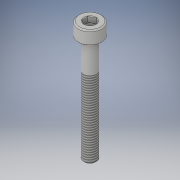
# Autodesk Inventor part: DIN-912 - M3x25(F)
Saved by Autodesk Inventor 2019 (Build 230136000, 136)
## iProperties
Created: 2023-04-07
Part Number: DIN-912 - M3x25(F)
Material: Generic
Catalog Web Link: www.cadenas.de
Description: DIN-912-Cylinder screw
Vendor: FESTO
Document SubType Name: Modeling
Designer: psAdmin
Manufacturer: FESTO
Mass: 0.238597 g
Surface Area: 3.40249 cm^2
Volume: 0.238597 cm^3
Density: 1 g/cm^3
Appearance: PSOLRGB-175-175-175
Category: PARTsolutions
Company: FESTO
Title: DIN-912 - M3x25(F)
Author: Cadenas PARTsolutions
Comments: Cylinder screw
PSOL_IDENT_0: {$CADENAS_DATA/23d-libs/festo/zyl_zubeh/d912/din_912.prj},178 {VTYP=3D},{NB=DIN-912 - M3x25(F)},{LIN
PSOL_IDENT_1: A=DIN-912 - M3x25(F)},{NN=DIN-912},{DATE=25.11.2021 14:13:45},{GEOMDATE=25.11.2021 14:12:35},{VERSIO
PSOL_IDENT_2: N=},{LINEID=160},{WBVAR=},{WBNUMERIC=}  {NB=DIN-912 - M3x25(F)},{LINA=DIN-912 - M3x25(F)},{KT=X},{ID
PSOL_IDENT_3: NR=},{GEW=M3},{DG=3.000},{P=0.500},{L=25.000},{B=18.000},{FORM=0},{GKD=2.387},{DK=5.500},{DADIN=3.60
PSOL_IDENT_4: 0},{DS=3.000},{E=2.870},{LF=0.510},{K=3.000},{R=0.120},{S=2.500},{T=1.300},{V=0.300},{DW=5.070},{W=1
PSOL_IDENT_5: .150},{NENN=M3x25},{DA=3.1},{BL=18}
NB: DIN-912 - M3x25(F)
NN: DIN-912
NT: Cylinder screw
NBSYN: DIN-912 - $NENN.(F)
LINA: DIN-912 - M3x25(F)
CATALOG: Festo
ROWDESC: M3x25
GEW: M3
DG: 3
P: 0.5
L: 25
B: 18
FORM: 0
GKD: 2.387
DK: 5.5
DADIN: 3.6
DS: 3
E: 2.87
LF: 0.51
K: 3
R: 0.12
S: 2.5
T: 1.3
V: 0.3
DW: 5.07
W: 1.15
SUPPLIER: FESTO
ARTICLENO: DIN-912 - M3x25(F)
BOMINFO: DIN-912 - M3x25(F)
CREATOR: CADENAS GmbH
Autodesk Inventor part; units mm, degrees
sketch "Sketch_1" plane through (0, 0, 0) normal (0, 0, 1) x (1, 0, 0)
  line L0 (0, -25) -> (0, 3)
  line L1 (0, 0.9783) -> (1.25, 1.7)
  line L2 (1.25, 1.7) -> (1.25, 2.8066)
  line L3 (1.25, 2.8066) -> (1.4434, 3)
  line L4 (1.4434, 3) -> (2.45, 3)
  line L5 (2.45, 3) -> (2.75, 2.7)
  line L6 (2.75, 2.7) -> (2.75, 0.075)
  line L7 (2.75, 0.075) -> (2.675, 0)
  line L8 (2.675, 0) -> (1.55, 0)
  line L9 (1.55, 0) -> (1.5, -0.51)
  line L10 (1.5, -0.51) -> (1.5, -24.6935)
  line L11 (1.5, -24.6935) -> (1.1935, -25)
  line L12 (1.1935, -25) -> (0, -25)
  line L13 (0, -25) -> (0, 0.9783)
  constraints: 28 end point
revolve "Revolution1" add sketch "Sketch_1" angle 360 about axis through (0, -25, 0) along (0, -1, 0)
thread "Thread1" size "M3x0.5" class "6g" standard "ISO Metric profile" length 17.6935
sketch "Sketch_2" plane through (0, 3, 0) normal (0, 1, 0) x (1, 0, 0)
  line L0 (-1.25, -0.7217) -> (0, -1.4434)
  line L1 (0, -1.4434) -> (1.25, -0.7217)
  line L2 (1.25, -0.7217) -> (1.25, 0.7217)
  line L3 (1.25, 0.7217) -> (0, 1.4434)
  line L4 (0, 1.4434) -> (-1.25, 0.7217)
  line L5 (-1.25, 0.7217) -> (-1.25, -0.7217)
  constraints: 12 end point
extrude "Extrusion1" cut sketch "Sketch_2" against normal blind 1.3
ref_plane "ANBAU_XY" through (0, 0, 0) normal (0, 1, 0) x (1, 0, 0)
ref_plane "ANBAU_YZ" through (0, 0, 0) normal (1, 0, 0) x (0, 0, -1)
ref_plane "ANBAU_ZX" through (0, 0, 0) normal (0, 0, -1) x (0, 1, 0)
ref_plane "Schraube_XY" through (0, 0, 0) normal (0, 1, 0) x (1, 0, 0)
ref_plane "Schraube_YZ" through (0, 0, 0) normal (1, 0, 0) x (0, 0, -1)
ref_plane "Schraube_ZX" through (0, 0, 0) normal (0, 0, -1) x (0, 1, 0)
ref_plane "insert_XY" through (0, 0, 0) normal (0, 1, 0) x (1, 0, 0)
ref_plane "insert_YZ" through (0, 0, 0) normal (1, 0, 0) x (0, 0, -1)
ref_plane "insert_ZX" through (0, 0, 0) normal (0, 0, -1) x (0, 1, 0)
ref_plane "schrauben_punkt_XY" through (0, -25, 0) normal (0, 1, 0) x (1, 0, 0)
ref_plane "schrauben_punkt_YZ" through (0, -25, 0) normal (1, 0, 0) x (0, 0, -1)
ref_plane "schrauben_punkt_ZX" through (0, -25, 0) normal (0, 0, -1) x (0, 1, 0)
body "Solid1"
